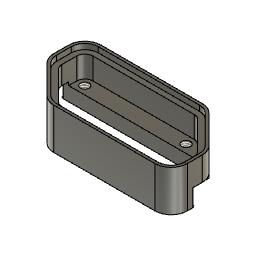
Collision Check - Practice (Autodesk Fusion 360 design; units mm, degrees)
Autodesk Fusion 360 part; units mm, degrees
sketch "Sketch1" plane through (0, 0, 0) normal (0, 0, 1) x (1, 0, 0) in component "Stock"
  line L0 (50.8, -25.4) -> (-50.8, -25.4)
  line L1 (-50.8, -25.4) -> (-50.8, 25.4)
  line L2 (-50.8, 25.4) -> (50.8, 25.4)
  line L3 (50.8, 25.4) -> (50.8, -25.4)
  line L4 (50.8, -25.4) -> (-50.8, 25.4) construction
  line L5 (-50.8, -25.4) -> (50.8, 25.4) construction
  dimension "d1" = 101.6
  dimension "d2" = 50.8
  constraint horizontal L0
  constraint perpendicular L0 L1
  constraint parallel L0 L2
  constraint parallel L1 L3
  constraint coincident L4 origin
  constraint coincident L5 origin
  measures "d1" distance of L1.end L2.end
  measures "d2" distance of L0.end L1.end
extrude "Extrude1" add sketch "Sketch1" along normal blind 19.05 and the other way blind 6.35 makes body 1 in component "Stock"
sketch "Sketch1 (2)" plane through (0, 0, 0) normal (0, 0, 1) x (1, 0, 0) in component "Part"
  line L0 (47.625, -22.225) -> (-47.625, -22.225)
  line L1 (-47.625, -22.225) -> (-47.625, 22.225)
  line L2 (-47.625, 22.225) -> (47.625, 22.225)
  line L3 (47.625, 22.225) -> (47.625, -22.225)
  line L4 (47.625, -22.225) -> (-47.625, 22.225) construction
  line L5 (-47.625, -22.225) -> (47.625, 22.225) construction
  dimension "d7" = 95.25
  dimension "d8" = 44.45
  constraint horizontal L0
  constraint perpendicular L0 L1
  constraint parallel L0 L2
  constraint parallel L1 L3
  constraint coincident L4 origin
  constraint coincident L5 origin
  measures "d7" distance of L1.end L2.end
  measures "d8" distance of L0.end L1.end
extrude "Extrude1'" add sketch "Sketch1 (2)" along normal blind 24.13 separate body makes body 2 in component "Part"
sketch "Sketch2" plane through (0, 0, 24.13) normal (0, 0, 1) x (-1, 0, 0) in component "Part"
  line L0 (-47.625, -22.225) -> (47.625, -22.225)
  line L1 (47.625, -22.225) -> (47.625, 22.225)
  line L2 (47.625, 22.225) -> (-47.625, 22.225)
  line L3 (-47.625, 22.225) -> (-47.625, -22.225)
  line L4 (47.625, 0) -> (25.4, -22.225) construction
  line L5 (-47.625, 0) -> (-25.4, 22.225) construction
  line L6 (47.625, 0) -> (25.4, 22.225)
  line L7 (-47.625, 0) -> (-25.4, -22.225)
  dimension "d11" = 45
  dimension "d12" = 45
  dimension "d19" = 45
  dimension "d20" = 45
  constraint midpoint L1 L4.start
  constraint coincident L0 L4.end
  constraint midpoint L3 L5.start
  constraint coincident L2 L5.end
  constraint coincident L2 L6.end
  constraint coincident L0 L7.end
  measures "d11" angle of L1 L4
  measures "d12" angle of L3 L5
  measures "d19" angle of L3 L7
  measures "d20" angle of L1 L6
extrude "Extrude2" cut sketch "Sketch2" against normal through all contours L0 L3 L7 | L1 L2 L6 bodies 2 in component "Part"
fillet "Fillet1" radius 9.525 6 edges at (-47.625, 0, 12.065) (-25.4, -22.225, 12.065) (47.625, -22.225, 12.065) (47.625, 0, 12.065) (25.4, 22.225, 12.065) (-47.625, 22.225, 12.065) on bodies 2 in component "Part"
sketch "Sketch3" plane through (0, 0, 24.13) normal (0, 0, 1) x (-1, 0, 0) in component "Part"
  arc A0 (38.1, -22.225) -> (47.625, -12.7) centre (38.1, -12.7) ccw
  line L0 (47.625, -12.7) -> (47.625, -3.9454)
  arc A1 (47.625, -3.9454) -> (44.8352, 2.7898) centre (38.1, -3.9454) ccw
  line L1 (44.8352, 2.7898) -> (28.1898, 19.4352)
  arc A2 (28.1898, 19.4352) -> (21.4546, 22.225) centre (21.4546, 12.7) ccw
  line L2 (21.4546, 22.225) -> (-38.1, 22.225)
  arc A3 (-38.1, 22.225) -> (-47.625, 12.7) centre (-38.1, 12.7) ccw
  line L3 (-47.625, 12.7) -> (-47.625, 3.9454)
  arc A4 (-47.625, 3.9454) -> (-44.8352, -2.7898) centre (-38.1, 3.9454) ccw
  line L4 (-44.8352, -2.7898) -> (-28.1898, -19.4352)
  arc A5 (-28.1898, -19.4352) -> (-21.4546, -22.225) centre (-21.4546, -12.7) ccw
  line L5 (-21.4546, -22.225) -> (38.1, -22.225)
  line L6 (46.0375, -12.7) -> (46.0375, -3.9454)
  arc A6 (46.0375, -3.9454) -> (43.7127, 1.6673) centre (38.1, -3.9454) ccw
  line L7 (43.7127, 1.6673) -> (27.0673, 18.3127)
  arc A7 (27.0673, 18.3127) -> (21.4546, 20.6375) centre (21.4546, 12.7) ccw
  line L8 (21.4546, 20.6375) -> (-38.1, 20.6375)
  arc A8 (-38.1, 20.6375) -> (-46.0375, 12.7) centre (-38.1, 12.7) ccw
  line L9 (-46.0375, 12.7) -> (-46.0375, 3.9454)
  arc A9 (-46.0375, 3.9454) -> (-43.7127, -1.6673) centre (-38.1, 3.9454) ccw
  line L10 (-43.7127, -1.6673) -> (-27.0673, -18.3127)
  arc A10 (-27.0673, -18.3127) -> (-21.4546, -20.6375) centre (-21.4546, -12.7) ccw
  line L11 (-21.4546, -20.6375) -> (38.1, -20.6375)
  arc A11 (38.1, -20.6375) -> (46.0375, -12.7) centre (38.1, -12.7) ccw
  dimension "d23" = -1.5875
extrude "Extrude3" cut sketch "Sketch3" against normal blind 3.175 contours L6 A6 L7 A7 L8 A8 L9 A9 L10 A10 L11 A11 bodies 2 in component "Part"
sketch "Sketch4" plane through (0, 0, 20.955) normal (0, 0, 1) x (-1, 0, 0) in component "Part"
  arc A0 (38.1, -20.6375) -> (46.0375, -12.7) centre (38.1, -12.7) ccw
  line L0 (46.0375, -12.7) -> (46.0375, -3.9454)
  arc A1 (46.0375, -3.9454) -> (43.7127, 1.6673) centre (38.1, -3.9454) ccw
  line L1 (43.7127, 1.6673) -> (27.0673, 18.3127)
  arc A2 (27.0673, 18.3127) -> (21.4546, 20.6375) centre (21.4546, 12.7) ccw
  line L2 (21.4546, 20.6375) -> (-38.1, 20.6375)
  arc A3 (-38.1, 20.6375) -> (-46.0375, 12.7) centre (-38.1, 12.7) ccw
  line L3 (-46.0375, 12.7) -> (-46.0375, 3.9454)
  arc A4 (-46.0375, 3.9454) -> (-43.7127, -1.6673) centre (-38.1, 3.9454) ccw
  line L4 (-43.7127, -1.6673) -> (-27.0673, -18.3127)
  arc A5 (-27.0673, -18.3127) -> (-21.4546, -20.6375) centre (-21.4546, -12.7) ccw
  line L5 (-21.4546, -20.6375) -> (38.1, -20.6375)
  line L6 (42.8625, -12.7) -> (42.8625, -3.9454)
  arc A6 (42.8625, -3.9454) -> (41.4676, -0.5778) centre (38.1, -3.9454) ccw
  line L7 (41.4676, -0.5778) -> (24.8222, 16.0676)
  arc A7 (24.8222, 16.0676) -> (21.4546, 17.4625) centre (21.4546, 12.7) ccw
  line L8 (21.4546, 17.4625) -> (-38.1, 17.4625)
  arc A8 (-38.1, 17.4625) -> (-42.8625, 12.7) centre (-38.1, 12.7) ccw
  line L9 (-42.8625, 12.7) -> (-42.8625, 3.9454)
  arc A9 (-42.8625, 3.9454) -> (-41.4676, 0.5778) centre (-38.1, 3.9454) ccw
  line L10 (-41.4676, 0.5778) -> (-24.8222, -16.0676)
  arc A10 (-24.8222, -16.0676) -> (-21.4546, -17.4625) centre (-21.4546, -12.7) ccw
  line L11 (-21.4546, -17.4625) -> (38.1, -17.4625)
  arc A11 (38.1, -17.4625) -> (42.8625, -12.7) centre (38.1, -12.7) ccw
  dimension "d24" = -3.175
extrude "Extrude4" cut sketch "Sketch4" against normal blind 12.7 contours L6 A6 L7 A7 L8 A8 L9 A9 L10 A10 L11 A11 bodies 2 in component "Part"
sketch "Sketch5" plane through (0, 0, 8.255) normal (0, 0, 1) x (-1, 0, 0) in component "Part"
  arc A0 (38.1, -17.4625) -> (42.8625, -12.7) centre (38.1, -12.7) ccw
  line L0 (42.8625, -12.7) -> (42.8625, -3.9454)
  arc A1 (42.8625, -3.9454) -> (41.4676, -0.5778) centre (38.1, -3.9454) ccw
  line L1 (41.4676, -0.5778) -> (24.8222, 16.0676)
  arc A2 (24.8222, 16.0676) -> (21.4546, 17.4625) centre (21.4546, 12.7) ccw
  line L2 (21.4546, 17.4625) -> (-38.1, 17.4625)
  arc A3 (-38.1, 17.4625) -> (-42.8625, 12.7) centre (-38.1, 12.7) ccw
  line L3 (-42.8625, 12.7) -> (-42.8625, 3.9454)
  arc A4 (-42.8625, 3.9454) -> (-41.4676, 0.5778) centre (-38.1, 3.9454) ccw
  line L4 (-41.4676, 0.5778) -> (-24.8222, -16.0676)
  arc A5 (-24.8222, -16.0676) -> (-21.4546, -17.4625) centre (-21.4546, -12.7) ccw
  line L5 (-21.4546, -17.4625) -> (38.1, -17.4625)
  point P0 (38.1, -12.7)
  point P1 (25.4, -12.7)
  point P2 (12.7, -12.7)
  point P3 (0, -12.7)
  point P4 (-12.7, -12.7)
  point P5 (25.4, 0)
  point P6 (12.7, 0)
  point P7 (-12.7, 0)
  point P8 (-25.4, 0)
  point P9 (12.7, 12.7)
  point P10 (0, 12.7)
  point P11 (-12.7, 12.7)
  point P12 (-25.4, 12.7)
  point P13 (-38.1, 12.7)
  point P14 (-21.4546, -12.7)
  point P15 (21.4546, 12.7)
  dimension "d27" = 12.7
  dimension "d28" = 12.7
  dimension "d29" = 12.7
  dimension "d30" = 12.7
  constraint coincident P0 A0.centre
  constraint coincident P13 A3.centre
  constraint horizontal P12 P13
  constraint horizontal P11 P12
  constraint horizontal P10 P11
  constraint horizontal P9 P10
  constraint vertical P8 P12
  constraint vertical P7 P11
  constraint vertical origin P10
  constraint vertical P6 P9
  constraint horizontal P5 P6
  constraint horizontal origin P6
  constraint horizontal origin P7
  constraint horizontal P7 P8
  constraint horizontal P0 P1
  constraint horizontal P1 P2
  constraint horizontal P2 P3
  constraint horizontal P3 P4
  constraint vertical P1 P5
  constraint vertical P2 P6
  constraint vertical P3 origin
  constraint vertical P4 P7
  constraint coincident P14 A5.centre
  constraint coincident P15 A2.centre
  measures "d27" distance of P12 P13
  measures "d28" distance of P11 P12
  measures "d29" distance of P9 P10
  measures "d30" distance of P5 P6
hole "Hole2" at (-38.1, 12.7, 8.255) at (21.4546, 12.7, 8.255) at (38.1, -12.7, 8.255) at (-21.4546, -12.7, 8.255) direction (0, 0, -1) diameter 5.1308 end through all bodies 2 in component "Part"
thread "Thread2" "ANSI Unified Screw Threads 0.25 1/4-20 UNC 1B" in component "Part"
sketch "Sketch6" plane through (0, 0, 0) normal (0, 0, -1) x (1, 0, 0) in component "Part"
  arc A0 (-47.625, -12.7) -> (-38.1, -22.225) centre (-38.1, -12.7) ccw
  line L0 (-38.1, -22.225) -> (21.4546, -22.225)
  arc A1 (21.4546, -22.225) -> (28.1898, -19.4352) centre (21.4546, -12.7) ccw
  line L1 (28.1898, -19.4352) -> (44.8352, -2.7898)
  arc A2 (44.8352, -2.7898) -> (47.625, 3.9454) centre (38.1, 3.9454) ccw
  line L2 (47.625, 3.9454) -> (47.625, 12.7)
  arc A3 (47.625, 12.7) -> (38.1, 22.225) centre (38.1, 12.7) ccw
  line L3 (38.1, 22.225) -> (-21.4546, 22.225)
  arc A4 (-21.4546, 22.225) -> (-28.1898, 19.4352) centre (-21.4546, 12.7) ccw
  line L4 (-28.1898, 19.4352) -> (-44.8352, 2.7898)
  arc A5 (-44.8352, 2.7898) -> (-47.625, -3.9454) centre (-38.1, -3.9454) ccw
  line L5 (-47.625, -3.9454) -> (-47.625, -12.7)
  line L6 (63.5, -7.9375) -> (-63.5, -7.9375)
  line L7 (-63.5, -7.9375) -> (-63.5, 7.9375)
  line L8 (-63.5, 7.9375) -> (63.5, 7.9375)
  line L9 (63.5, 7.9375) -> (63.5, -7.9375)
  line L10 (63.5, -7.9375) -> (-63.5, 7.9375) construction
  line L11 (-63.5, -7.9375) -> (63.5, 7.9375) construction
  circle A6 centre (38.1, 12.7) radius 2.5591
  circle A7 centre (-38.1, -12.7) radius 2.5591
  circle A8 centre (21.4546, -12.7) radius 2.5591
  circle A9 centre (-21.4546, 12.7) radius 2.5591
  dimension "d37" = 127
  dimension "d38" = 15.875
  constraint horizontal L6
  constraint perpendicular L6 L7
  constraint parallel L6 L8
  constraint parallel L7 L9
  constraint coincident L10 origin
  constraint coincident L11 origin
  measures "d37" distance of L7.end L8.end
  measures "d38" distance of L6.end L7.end
extrude "Extrude5" cut sketch "Sketch6" against normal blind 10.16 contours L1 A2 L2 L4 A5 L5 L6 L8 bodies 2 in component "Part"
fillet "Fillet2" radius 1.5875 4 edges at (-39.6875, -7.9375, 5.08) (-47.625, 7.9375, 5.08) (47.625, -7.9375, 5.08) (39.6875, 7.9375, 5.08) on bodies 2 in component "Part"
component "Stock" placed x (1, 0, 0) y (0, 1, 0) z (0, 0, 1) at (0, 0, 0)
component "Part" placed x (1, 0, 0) y (0, 1, 0) z (0, 0, 1) at (0, 0, 0)
equation "d28 = d27"
equation "d29 = d27"
equation "d30 = d27"
